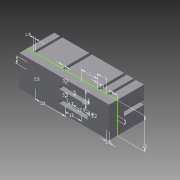
# Autodesk Inventor part: Spirulina_prototype
Saved by Autodesk Inventor 2015 (Build 190159000, 159)
## iProperties
Created: 2015-05-18
Part Number: Spirulina_prototype
Material: Generic
Document SubType Name: Modeling
Designer: Openlab
Density: 1 g/cm^3
Appearance: Default
Author: Openlab
Autodesk Inventor part; units mm, degrees
ref_plane "YZ Plane" through (0, 0, 0) normal (1, 0, 0) x (0, 1, 0)
ref_plane "XZ Plane" through (0, 0, 0) normal (0, 1, 0) x (-1, 0, 0)
ref_plane "XY Plane" through (0, 0, 0) normal (0, 0, 1) x (1, 0, 0)
sketch "Sketch1" plane through (0, 0, 0) normal (0, 1, 0) x (-1, 0, 0)
  line L0 (73.75, -5.35) -> (61.25, -5.35)
  line L1 (61.25, -5.35) -> (61.25, -17.85)
  line L2 (61.25, -17.85) -> (73.75, -17.85)
  line L3 (73.75, -17.85) -> (73.75, -5.35)
  line L4 (107.5984, -0.1) -> (40.7, -0.1)
  line L5 (40.7, -23.1) -> (107.5984, -23.1)
  line L6 (77.3838, -11.6) -> (49.3838, -11.6) construction
  line L7 (67.5, -2.25) -> (67.5, -23.25) construction
  line L8 (101.5, -0.1) -> (101.5, -23.1)
  line L9 (103.3, -23.1) -> (103.3, -0.1)
  line L10 (81.5, -9.1) -> (107.5984, -9.1)
  line L11 (107.5984, -14.1) -> (81.5, -14.1)
  line L12 (48.5, -23.1) -> (48.5, -0.1)
  line L13 (46.7, -0.1) -> (46.7, -23.1)
  line L14 (53.5, -10.1) -> (40.7, -10.1)
  line L15 (53.5, -13.1) -> (40.7, -13.1)
  line L16 (101.5, -15.5) -> (100, -15.5)
  line L17 (100, -15.5) -> (100, -7.7)
  line L18 (100, -7.7) -> (101.5, -7.7)
  line L19 (79.5, -0.1) -> (79.5, -23.1)
  line L20 (81.5, -23.1) -> (81.5, -0.1)
  line L21 (55.5, -0.1) -> (55.5, -23.1)
  line L22 (53.5, -23.1) -> (53.5, -0.1)
  line L23 (79.5, -13.1) -> (73.75, -13.1)
  line L24 (73.75, -10.1) -> (79.5, -10.1)
  line L25 (61.25, -13.1) -> (55.5, -13.1)
  line L26 (55.5, -10.1) -> (61.25, -10.1)
  line L27 (73.75, -17.85) -> (77.95, -17.85)
  line L28 (77.95, -17.85) -> (77.95, -14.65)
  line L29 (77.95, -14.65) -> (73.75, -14.65)
  line L30 (73.75, -14.65) -> (61.25, -14.65)
  line L31 (56.65, -14.65) -> (56.65, -17.85)
  line L32 (56.65, -17.85) -> (59.85, -17.85)
  line L33 (59.85, -14.65) -> (56.65, -14.65)
  line L34 (59.85, -5.35) -> (56.65, -5.35)
  line L35 (56.65, -5.35) -> (56.65, -8.55)
  line L36 (56.65, -8.55) -> (59.85, -8.55)
  line L37 (61.25, -8.55) -> (73.75, -8.55)
  line L38 (77.95, -8.55) -> (77.95, -5.35)
  line L39 (73.75, -5.35) -> (77.95, -5.35)
  line L40 (77.95, -8.55) -> (73.75, -8.55)
  line L41 (59.85, -17.85) -> (59.85, -14.65)
  line L42 (59.85, -8.55) -> (59.85, -5.35)
  line L43 (61.25, -17.85) -> (59.85, -17.85)
  line L44 (61.25, -14.65) -> (59.85, -14.65)
  line L45 (61.25, -8.55) -> (59.85, -8.55)
  line L46 (61.25, -5.35) -> (59.85, -5.35)
  line L47 (40.7, -23.1) -> (40.7, -0.1)
  line L48 (107.5984, -23.1) -> (107.5984, -0.1)
  point P0 (103.3, -9.1)
  point P1 (101.5, -9.1)
  point P2 (103.3, -14.1)
  point P3 (101.5, -14.1)
  point P4 (48.5, -10.1)
  point P5 (46.7, -10.1)
  point P6 (48.5, -13.1)
  point P7 (46.7, -13.1)
  point P8 (67.5, -11.6)
  point P9 (100, -9.1)
  point P10 (100, -14.1)
  dimension "d0" = 12.5
  dimension "d1" = 12.5
  dimension "d7" = 1.8
  dimension "d12" = 5
  dimension "d18" = 1.8
  dimension "d39" = 1.5
  dimension "d43" = 2
  dimension "d45" = 2
  dimension "d52" = 12
  dimension "d57" = 12
  dimension "d62" = 3
  dimension "d63" = 3
  dimension "d67" = 22
  dimension "d71" = 7
  dimension "d76" = 4.2
  dimension "d77" = 3.2
  dimension "d78" = 3.2
  dimension "d79" = 1.4
  dimension "d80" = 3.2
  dimension "d91" = 6
  dimension "d92" = 3
  dimension "d95" = 23
  constraints: 94 end point, 56 point on line, 14 perpendicular, 11 vertical, 8 horizontal, 8 parallel, 29 other
  measures "d0" distance of L2.end L1.end
  measures "d1" distance of L0.end L1.end
  measures "d7" distance between parallel lines of L9 L8
  measures "d12" distance between parallel lines of L11 L10
  measures "d18" distance between parallel lines of L13 L12
  measures "d39" distance of L16.start L16.end
  measures "d43" distance between parallel lines of L20 L19
  measures "d45" distance between parallel lines of L22 L21
  measures "d52" distance between parallel lines of L21 L7
  measures "d57" distance between parallel lines of L19 L7
  measures "d62" distance between parallel lines of L24 L23
  measures "d63" distance between parallel lines of L26 L25
  measures "d67" distance between parallel lines of L8 L19
  measures "d71" distance between parallel lines of L12 L21
  measures "d76" distance of L2.end L27.end
  measures "d77" distance of L27.end L28.end
  measures "d78" distance of L38.start L38.end
  measures "d79" distance between parallel lines of L41 L1
  measures "d80" distance of L31.end L32.end
  measures "d91" distance between parallel lines of L47 L13
  measures "d92" distance between parallel lines of L14 L15
  measures "d95" distance of L47.start L47.end
extrude "Extrusion11" add sketch "Sketch1" against normal blind 3 contours L3 L37 L1 L0 | L1 L45 L42 L46 | L3 L2 L1 L30 | L1 L43 L41 L44
extrude "Extrusion10" add sketch "Sketch1" against normal blind 6 separate body contours L0 L46 L34 L35 L36 L45 L1 L26 L21 L4 L19 L24 L3 L40 L38 L39 | L3 L30 L1 L37 | L24 L19 L23 L3 | L1 L25 L21 L26 | L23 L19 L5 L21 L25 L1 L44 L33 L31 L32 L43 L2 L27 L28 L29 L3 | L19 L4 L20 L5 | L21 L5 L22 L4 | L4 L8 L18 L17 L10 L20 | L22 L14 L12 L4 | L20 L11 L17 L16 L8 L5 | L4 L9 L10 L8 | L10 L17 L11 L20 | L5 L12 L15 L22 | L12 L14 L13 L4 | L22 L15 L12 L14 | L8 L11 L9 L5 | L4 L48 L10 L9 | L8 L10 L17 L18 | L10 L8 L11 L17 | L5 L13 L15 L12 | L13 L14 L47 L4 | L12 L15 L13 L14 | L9 L11 L48 L5 | L16 L17 L11 L8 | L10 L48 L11 L9 | L9 L11 L8 L10 | L5 L47 L15 L13 | L13 L15 L47 L14
extrude "Extrusion15" add sketch "Sketch1" along normal blind 5 contours L0 L46 L34 L35 L36 L45 L1 L26 L21 L4 L19 L24 L3 L40 L38 L39 | L24 L19 L23 L3 | L1 L25 L21 L26 | L23 L19 L5 L21 L25 L1 L44 L33 L31 L32 L43 L2 L27 L28 L29 L3 | L4 L8 L18 L17 L10 L20 | L22 L14 L12 L4 | L20 L11 L17 L16 L8 L5 | L10 L17 L11 L20 | L5 L12 L15 L22 | L22 L15 L12 L14 | L4 L48 L10 L9 | L8 L10 L17 L18 | L10 L8 L11 L17 | L13 L14 L47 L4 | L9 L11 L48 L5 | L16 L17 L11 L8 | L10 L48 L11 L9 | L5 L47 L15 L13 | L13 L15 L47 L14
extrude "Extrusion14" add sketch "Sketch1" along normal blind 3.5 contours L3 L37 L1 L0 | L3 L30 L1 L37 | L3 L2 L1 L30
extrude "Extrusion16" add sketch "Sketch1" along normal blind 20 contours L0 L46 L34 L35 L36 L45 L1 L26 L21 L4 L19 L24 L3 L40 L38 L39 | L1 L45 L42 L46 | L23 L19 L5 L21 L25 L1 L44 L33 L31 L32 L43 L2 L27 L28 L29 L3 | L1 L43 L41 L44 | L4 L8 L18 L17 L10 L20 | L22 L14 L12 L4 | L20 L11 L17 L16 L8 L5 | L5 L12 L15 L22 | L4 L48 L10 L9 | L13 L14 L47 L4 | L9 L11 L48 L5 | L5 L47 L15 L13
body "Solid3"
